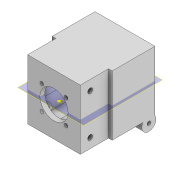
# Autodesk Inventor part: StepperMotorHolder
Saved by Autodesk Inventor 2022 (Build 260153000, 153)
## iProperties
Created: 2022-10-20
Part Number: StepperMotorHolder
Material: Generic
Document SubType Name: Modeling
Designer: MVeszpremi
Density: 1 g/cm^3
Appearance: Default
Author: MVeszpremi
Autodesk Inventor part; units mm, degrees
ref_plane "YZ Plane" through (0, 0, 0) normal (1, 0, 0) x (0, 1, 0)
ref_plane "XZ Plane" through (0, 0, 0) normal (0, 1, 0) x (-1, 0, 0)
ref_plane "XY Plane" through (0, 0, 0) normal (0, 0, 1) x (1, 0, 0)
sketch "Sketch1" plane through (0, 0, 0) normal (0, 0, 1) x (1, 0, 0)
  line L0 (-21.5, -21.5) -> (21.5, -21.5)
  line L1 (21.5, -21.5) -> (21.5, 21.5)
  line L2 (21.5, 21.5) -> (-21.5, 21.5)
  line L3 (-21.5, 21.5) -> (-21.5, -21.5)
  line L4 (-21.5, -21.5) -> (21.5, 21.5) construction
  line L5 (21.5, -21.5) -> (-21.5, 21.5) construction
  circle A0 centre (0, 0) radius 18.5
  circle A1 centre (0, 0) radius 11.5
  circle A2 centre (0, 0) radius 14
  circle A3 centre (-9.8995, 9.8995) radius 1.5
  circle A4 centre (-9.8995, -9.8995) radius 1.5
  circle A5 centre (9.8995, -9.8995) radius 1.5
  circle A6 centre (9.8995, 9.8995) radius 1.5
  line L6 (0, 0) -> (0, 21.5)
  line L7 (-24.5, 24.5) -> (24.5, 24.5)
  line L8 (24.5, 24.5) -> (24.5, -24.5)
  line L9 (24.5, -24.5) -> (-24.5, -24.5)
  line L10 (-24.5, -24.5) -> (-24.5, 24.5)
  line L11 (-24.5, 24.5) -> (24.5, -24.5) construction
  line L12 (24.5, 24.5) -> (-24.5, -24.5) construction
  dimension "d4" = 28
  dimension "d0" = 43
  dimension "d1" = 43
  dimension "d2" = 37
  dimension "d3" = 23
  dimension "d5" = 3
  dimension "d8" = 360
  dimension "d10" = 3
  dimension "d11" = 3
  constraints: 26 end point, 6 centre point, 5 midpoint, 4 parallel, 3 coincident, 2 horizontal, 2 perpendicular, 1 point on line, 12 other
  measures "d0" distance of L1.end L2.end
  measures "d1" distance of L2.end L0.start
  measures "d2" diameter of A0
  measures "d3" diameter of A1
  measures "d5" diameter of A3
  measures "d10" distance between parallel lines of L10 L3
  measures "d11" distance between parallel lines of L9 L0
extrude "Extrusion1" add sketch "Sketch1" along normal blind 5 and the other way blind 30 contours L7 L8 L9 L10
extrude "Extrusion2" add sketch "Sketch1" along normal blind 24 contours L3 L2 L1 L0
sketch "Sketch2" plane through (0, 0, 24) normal (0, 0, 1) x (1, 0, 0)
  circle A0 centre (0, 0) radius 11.5 projected
  circle A1 centre (0, 0) radius 14 projected
  circle A2 centre (9.8995, 9.8995) radius 1.5 projected
  circle A3 centre (9.8995, -9.8995) radius 1.5 projected
  circle A4 centre (-9.8995, -9.8995) radius 1.5 projected
  circle A5 centre (-9.8995, 9.8995) radius 1.5 projected
  circle A6 centre (0, 0) radius 18.5 projected
  line L0 (-21.5, 21.5) -> (-21.5, -21.5) projected
  line L1 (-21.5, -21.5) -> (21.5, -21.5) projected
  line L2 (21.5, -21.5) -> (21.5, 21.5) projected
  line L3 (21.5, 21.5) -> (-21.5, 21.5) projected
  circle A7 centre (0, 0) radius 18.5 projected
  line L4 (24.5, -24.5) -> (-24.5, -24.5) projected
  line L5 (24.5, 24.5) -> (24.5, -24.5) projected
  line L6 (-24.5, 24.5) -> (24.5, 24.5) projected
  line L7 (-24.5, -24.5) -> (-24.5, 24.5) projected
  line L8 (21.5, -21.5) -> (21.5, 21.5) projected
  line L9 (-21.5, -21.5) -> (21.5, -21.5) projected
  line L10 (-21.5, 21.5) -> (-21.5, -21.5) projected
  line L11 (21.5, 21.5) -> (-21.5, 21.5) projected
extrude "Extrusion3" add sketch "Sketch2" along normal blind 4 contours A1 A3 A4 A5 A2 | A6 | L3 L2 L1 L0
chamfer "Chamfer1" distance 2 angle 45 4 edges at (21.5, 21.5, -15) (-21.5, 21.5, -15) (-21.5, -21.5, -15) (21.5, -21.5, -15)
ref_plane "Work Plane1" through (-20.5, 0, -30) normal (0, 1, 0) x (1, 0, 0)
ref_plane "Work Plane3" through (24.5, -24.5, -20) normal (1, 0, 0) x (0, 0, -1)
sketch "Sketch8" plane through (24.5, -24.5, -20) normal (1, 0, 0) x (0, 0, -1)
  circle A0 centre (5, -3) radius 1.5
  circle A1 centre (5, -3) radius 5.831
  line L0 (10, 0) -> (-25, 0) projected
  line L1 (10, 49) -> (10, 0) projected
  point P0 (-20, 24.5)
  point P1 (10, 45)
  dimension "d70" = 3
  dimension "d76" = 3
  dimension "d77" = 5
  constraints: 1 centre point, 1 coincident, 3 other
  measures "d70" diameter of A0
  measures "d76" distance from line of L0 A0.centre
  measures "d77" distance from line of L1 A0.centre
extrude "Extrusion8" add sketch "Sketch8" against normal up to surface (49 mm away)
sketch "Sketch9" plane through (21.5, -21.5, 5) normal (1, 0, 0) x (0, 0, -1)
  circle A0 centre (-15, 38) radius 2
  line L0 (0, 43) -> (-23, 43) projected
  line L1 (-23, 0) -> (-23, 43) projected
  point P0 (5, 21.5)
  dimension "d79" = 5
  dimension "d80" = 8
  dimension "d81" = 4
  constraints: 1 centre point
  measures "d79" distance from line of L0 A0.centre
  measures "d80" distance from line of L1 A0.centre
  measures "d81" diameter of A0
extrude "Extrusion9" cut sketch "Sketch9" against normal blind 10
sketch "Sketch10" plane through (0, 0, 0) normal (0, 0, -1) x (-1, 0, 0)
  circle A0 centre (0, 0) radius 18.5 projected
  line L0 (21.5, 21.5) -> (-21.5, 21.5) projected
  line L1 (-18.5, 0) -> (18.5, 0)
  line L2 (18.5, 0) -> (18.5, 21.5)
  line L3 (18.5, 21.5) -> (-18.5, 21.5)
  line L4 (-18.5, 21.5) -> (-18.5, 0)
  line L5 (-21.5, 21.5) -> (21.5, 21.5) projected
  line L6 (5, -21.5) -> (-5, -21.5)
  line L7 (-5, -21.5) -> (-5, 21.5)
  line L8 (-5, 21.5) -> (5, 21.5)
  line L9 (5, 21.5) -> (5, -21.5)
  line L10 (5, -21.5) -> (-5, 21.5) construction
  line L11 (-5, -21.5) -> (5, 21.5) construction
  line L12 (18.5, -7.5) -> (-18.5, -7.5)
  line L13 (-18.5, -7.5) -> (-18.5, 7.5)
  line L14 (-18.5, 7.5) -> (18.5, 7.5)
  line L15 (18.5, 7.5) -> (18.5, -7.5)
  line L16 (18.5, -7.5) -> (-18.5, 7.5) construction
  line L17 (-18.5, -7.5) -> (18.5, 7.5) construction
  point P0 (5, 17.8115)
  point P1 (-5, 17.8115)
  point P2 (16.9115, 7.5)
  point P3 (18.5, 7.5)
  point P4 (-16.9115, 7.5)
  dimension "d94" = 10
  dimension "d95" = 15
  constraints: 32 end point, 6 parallel, 4 midpoint, 3 horizontal, 3 perpendicular, 3 point on line, 2 point on circle
  measures "d94" distance between parallel lines of L9 L7
  measures "d95" distance between parallel lines of L12 L14
sketch "Sketch11" plane through (0, 0, 5) normal (0, 0, 1) x (1, 0, 0)
  line L0 (-21.5, 21.5) -> (21.5, 21.5) projected
  line L1 (24.5, 24.5) -> (-24.5, 24.5) projected
  line L2 (-21.5, 21.5) -> (21.5, 21.5)
  line L3 (21.5, 21.5) -> (21.5, 24.5)
  line L4 (21.5, 24.5) -> (-21.5, 24.5)
  line L5 (-21.5, 24.5) -> (-21.5, 21.5)
  point P0 (0, 0)
  constraints: 8 end point, 2 parallel, 1 horizontal, 1 perpendicular, 1 point on line
extrude "Extrusion10" add sketch "Sketch11" along normal up to surface (23 mm away)
extrude "Extrusion11" cut sketch "Sketch10" against normal up to surface (24 mm away) contours A0 L9 L0 L2 L14 | A0 L14 L4 L0 L7
sketch "Sketch12" plane through (18.5, 0, 0) normal (-1, 0, 0) x (0, 0, 1)
  circle A0 centre (20, 16.5) radius 2 projected
  line L0 (19.9658, 20.6856) -> (23.6078, 18.6225)
  line L1 (23.6078, 18.6225) -> (23.642, 14.4368)
  line L2 (23.642, 14.4368) -> (20.0342, 12.3144)
  line L3 (20.0342, 12.3144) -> (16.3922, 14.3775)
  line L4 (16.3922, 14.3775) -> (16.358, 18.5632)
  line L5 (16.358, 18.5632) -> (19.9658, 20.6856)
  circle A1 centre (20, 16.5) radius 6
  point P0 (0, 0)
  dimension "d88" = 7.25
  dimension "d89" = 12
  constraints: 12 end point, 2 coincident, 1 centre point, 13 other
  measures "d88" distance between parallel lines of L1 L4
  measures "d89" diameter of A1
extrude "Extrusion12" add sketch "Sketch12" along normal blind 3 contours A1
mirror "Mirror2" about plane through (0, 0, 0) normal (1, 0, 0) of "Extrusion12", "Extrusion9"
sketch "Sketch13" plane through (0, 0, 24) normal (0, 0, -1) x (-1, 0, 0)
  point P0 (0, 0)
mirror "Mirror3" about plane through (0, 0, 0) normal (0, 1, 0) of "Extrusion12", "Extrusion9", "Mirror2", "Extrusion10", "Extrusion11"
ref_plane "Work Plane4" through (0, 0, 0) normal (0, 1, 0) x (-1, 0, 0)
body "Solid1"
